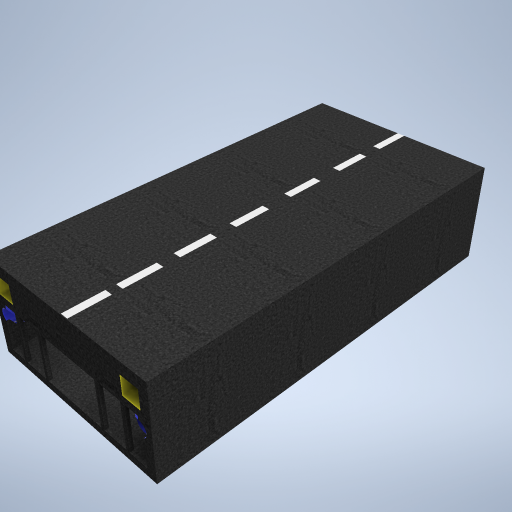
# Autodesk Inventor part: PLASTIC ROAD
Saved by Autodesk Inventor 2024 (Build 280153020, 153B)
## iProperties
Created: 2024-05-01
Part Number: PLASTIC ROAD
Material: Generic
Document SubType Name: Modeling
Designer: c7473124
Density: 1 g/cm^3
Appearance: Asphalt 2
Author: c7473124
Autodesk Inventor part; units mm, degrees
ref_plane "YZ Plane" through (0, 0, 0) normal (1, 0, 0) x (0, 1, 0)
ref_plane "XZ Plane" through (0, 0, 0) normal (0, 1, 0) x (-1, 0, 0)
ref_plane "XY Plane" through (0, 0, 0) normal (0, 0, 1) x (1, 0, 0)
sketch "Sketch1" plane through (0, 0, 0) normal (0, 0, 1) x (1, 0, 0)
  line L0 (0, 0) -> (1000, 0)
  line L1 (1000, 0) -> (1000, 500)
  line L2 (1000, 500) -> (0, 500)
  line L3 (0, 500) -> (0, 0)
  dimension "d0" = 1000
  dimension "d1" = 500
  constraints: 8 end point, 2 parallel, 1 horizontal, 1 perpendicular
  measures "d0" distance of L2.end L1.end
  measures "d1" distance of L1.end L0.end
extrude "Extrusion1" add sketch "Sketch1" along normal blind 2000
sketch "Sketch2" plane through (0, 0, 2000) normal (0, 0, 1) x (1, 0, 0)
  line L0 (947.5986, 433.5558) -> (847.5986, 433.5558)
  line L1 (847.5986, 433.5558) -> (847.5986, 333.5558)
  line L2 (847.5986, 333.5558) -> (947.5986, 333.5558)
  line L3 (947.5986, 333.5558) -> (947.5986, 433.5558)
  point P0 (0, 0)
  dimension "d4" = 100
  dimension "d5" = 100
  constraints: 8 end point, 2 parallel, 1 horizontal, 1 perpendicular
  measures "d4" distance of L2.end L1.end
  measures "d5" distance of L1.end L0.end
extrude "Extrusion2" cut sketch "Sketch2" against normal through all
sketch "Sketch3" plane through (0, 0, 2000) normal (0, 0, 1) x (1, 0, 0)
  line L0 (43.9995, 435.7022) -> (143.9995, 435.7022)
  line L1 (143.9995, 435.7022) -> (143.9995, 335.7022)
  line L2 (143.9995, 335.7022) -> (43.9995, 335.7022)
  line L3 (43.9995, 335.7022) -> (43.9995, 435.7022)
  point P0 (0, 0)
  dimension "d8" = 100
  dimension "d9" = 100
  constraints: 8 end point, 2 parallel, 1 horizontal, 1 perpendicular
  measures "d8" distance of L1.end L2.end
  measures "d9" distance of L0.end L1.end
extrude "Extrusion3" cut sketch "Sketch3" against normal through all
sketch "Sketch4" plane through (0, 0, 2000) normal (0, 0, 1) x (1, 0, 0)
  line L0 (50.4384, 294.0453) -> (949.7449, 294.0453)
  line L1 (949.7449, 294.0453) -> (949.7449, 42.9263)
  line L2 (949.7449, 42.9263) -> (50.4384, 42.9263)
  line L3 (50.4384, 42.9263) -> (50.4384, 294.0453)
  point P0 (0, 0)
  constraints: 8 end point, 2 parallel, 1 horizontal, 1 perpendicular
extrude "Extrusion4" cut sketch "Sketch4" against normal through all
sketch "Sketch5" plane through (50.4384, 42.9263, 2000) normal (1, 0, 0) x (0, 0, -1)
  line L0 (0, 251.119) -> (2000, 251.119) projected
  line L1 (2000, 251.119) -> (0, 251.119)
  line L2 (0, 251.119) -> (0, 171.119)
  line L3 (0, 171.119) -> (2000, 171.119)
  line L4 (2000, 171.119) -> (2000, 251.119)
  point P0 (2000, -42.9263)
  dimension "d14" = 2000
  dimension "d15" = 80
  constraints: 8 end point, 2 parallel, 1 horizontal, 1 perpendicular
  measures "d14" distance of L3.end L2.end
  measures "d15" distance of L2.end L1.end
extrude "Extrusion5" add sketch "Sketch5" along normal blind 70.5
sketch "Sketch6" plane through (0, 0, 2000) normal (0, 0, 1) x (1, 0, 0)
  line L0 (120.9384, 214.0453) -> (50.4384, 214.0453)
  line L1 (50.4384, 214.0453) -> (50.4384, 294.0453)
  line L2 (50.4384, 294.0453) -> (120.9384, 294.0453)
  line L3 (120.9384, 294.0453) -> (120.9384, 214.0453)
  point P0 (0, 0)
  constraints: 8 end point, 2 parallel, 1 horizontal, 1 perpendicular
extrude "Extrusion6" cut sketch "Sketch6" against normal through all
sketch "Sketch7" plane through (50.4384, 42.9263, 2000) normal (1, 0, 0) x (0, 0, -1)
  line L0 (0, 251.119) -> (2000, 251.119) projected
  line L1 (2000, 251.119) -> (0, 251.119)
  line L2 (0, 251.119) -> (0, 141.119)
  line L3 (0, 141.119) -> (2000, 141.119)
  line L4 (2000, 141.119) -> (2000, 251.119)
  point P0 (2000, -42.9263)
  dimension "d20" = 2000
  dimension "d21" = 110
  constraints: 8 end point, 2 parallel, 1 horizontal, 1 perpendicular
  measures "d20" distance of L3.end L2.end
  measures "d21" distance of L2.end L1.end
extrude "Extrusion7" add sketch "Sketch7" along normal blind 72
fillet "Fillet1" radius 50 3 edges at (122.4384, 239.0453, 2000) (86.4384, 184.0453, 2000) (122.4384, 184.0453, 1000)
sketch "Sketch8" plane through (0, 0, 2000) normal (0, 0, 1) x (1, 0, 0)
  line L0 (122.4384, 234.0453) -> (72.4384, 234.0453) projected
  circle A0 centre (72.4384, 234.0453) radius 40.25
  point P0 (0, 0)
  dimension "d25" = 80.5
  constraints: 1 centre point
  measures "d25" diameter of A0
extrude "Extrusion8" cut sketch "Sketch8" against normal through all
sketch "Sketch9" plane through (949.7449, 42.9263, 2000) normal (-1, 0, 0) x (0, 0, 1)
  line L0 (-50, 251.119) -> (-2000, 251.119) projected
  line L1 (-2000, 251.119) -> (0, 251.119)
  line L2 (0, 251.119) -> (0, 141.119)
  line L3 (0, 141.119) -> (-2000, 141.119)
  line L4 (-2000, 141.119) -> (-2000, 251.119)
  point P0 (-2000, -42.9263)
  dimension "d28" = 2000
  dimension "d29" = 110
  constraints: 8 end point, 2 parallel, 1 horizontal, 1 perpendicular
  measures "d28" distance of L2.end L3.end
  measures "d29" distance of L1.end L2.end
extrude "Extrusion9" add sketch "Sketch9" along normal blind 72
fillet "Fillet2" radius 50 3 edges at (877.7449, 239.0453, 2000) (913.7449, 184.0453, 2000) (877.7449, 184.0453, 1000)
sketch "Sketch10" plane through (0, 0, 2000) normal (0, 0, 1) x (1, 0, 0)
  line L0 (927.7449, 234.0453) -> (927.7449, 294.0453) projected
  circle A0 centre (927.7449, 234.0453) radius 41
  point P0 (0, 0)
  dimension "d33" = 82
  constraints: 1 centre point
  measures "d33" diameter of A0
extrude "Extrusion10" cut sketch "Sketch10" against normal through all
sketch "Sketch11" plane through (50.4384, 42.9263, 2000) normal (0, 1, 0) x (1, 0, 0)
  line L0 (93.5611, 0) -> (93.5611, 2000) projected
  line L1 (93.5611, 2000) -> (113.5611, 2000)
  line L2 (113.5611, 2000) -> (113.5611, 1980)
  line L3 (113.5611, 1980) -> (93.5611, 1980)
  line L4 (93.5611, 1980) -> (93.5611, 2000)
  point P0 (-50.4384, 2000)
  dimension "d36" = 20
  dimension "d37" = 20
  constraints: 8 end point, 2 parallel, 1 horizontal, 1 perpendicular
  measures "d36" distance of L2.end L3.end
  measures "d37" distance of L1.end L2.end
extrude "Extrusion11" add sketch "Sketch11" along normal through all
sketch "Sketch12" plane through (50.4384, 42.9263, 2000) normal (0, 1, 0) x (1, 0, 0)
  line L0 (797.1601, 0) -> (797.1601, 2000) projected
  line L1 (797.1601, 2000) -> (777.1601, 2000)
  line L2 (777.1601, 2000) -> (777.1601, 1980)
  line L3 (777.1601, 1980) -> (797.1601, 1980)
  line L4 (797.1601, 1980) -> (797.1601, 2000)
  point P0 (-50.4384, 2000)
  dimension "d40" = 20
  dimension "d41" = 20
  constraints: 8 end point, 2 parallel, 1 horizontal, 1 perpendicular
  measures "d40" distance of L3.end L2.end
  measures "d41" distance of L2.end L1.end
extrude "Extrusion12" add sketch "Sketch12" along normal through all
sketch "Sketch13" plane through (50.4384, 42.9263, 2000) normal (0, 1, 0) x (1, 0, 0)
  line L0 (777.1601, 2000) -> (113.5611, 2000) projected
  line L1 (258.2536, 2000) -> (278.2536, 2000)
  line L2 (278.2536, 2000) -> (278.2536, 1980)
  line L3 (278.2536, 1980) -> (258.2536, 1980)
  line L4 (258.2536, 1980) -> (258.2536, 2000)
  point P0 (-50.4384, 2000)
  dimension "d44" = 20
  dimension "d45" = 20
  constraints: 8 end point, 2 parallel, 1 horizontal, 1 perpendicular, 1 point on line
  measures "d44" distance of L2.end L3.end
  measures "d45" distance of L1.end L2.end
extrude "Extrusion13" add sketch "Sketch13" along normal through all
sketch "Sketch14" plane through (50.4384, 42.9263, 2000) normal (0, 1, 0) x (1, 0, 0)
  line L0 (278.2536, 2000) -> (777.1601, 2000) projected
  line L1 (651.9226, 2000) -> (631.9226, 2000)
  line L2 (631.9226, 2000) -> (631.9226, 1980)
  line L3 (631.9226, 1980) -> (651.9226, 1980)
  line L4 (651.9226, 1980) -> (651.9226, 2000)
  point P0 (-50.4384, 2000)
  dimension "d48" = 20
  dimension "d49" = 20
  constraints: 8 end point, 2 parallel, 1 horizontal, 1 perpendicular, 1 point on line
  measures "d48" distance of L3.end L2.end
  measures "d49" distance of L2.end L1.end
extrude "Extrusion14" add sketch "Sketch14" along normal through all
sketch "Sketch15" plane through (50.4384, 42.9263, 2000) normal (0, 1, 0) x (1, 0, 0)
  line L0 (93.5611, 0) -> (93.5611, 2000) projected
  line L1 (93.5611, 0) -> (113.5611, 0)
  line L2 (113.5611, 0) -> (113.5611, 20)
  line L3 (113.5611, 20) -> (93.5611, 20)
  line L4 (93.5611, 20) -> (93.5611, 0)
  point P0 (-50.4384, 2000)
  dimension "d52" = 20
  dimension "d53" = 20
  constraints: 8 end point, 2 parallel, 1 horizontal, 1 perpendicular
  measures "d52" distance of L3.end L2.end
  measures "d53" distance of L2.end L1.end
extrude "Extrusion15" add sketch "Sketch15" along normal through all
sketch "Sketch16" plane through (949.7449, 42.9263, 2000) normal (0, 1, 0) x (1, 0, 0)
  line L0 (-102.1463, 0) -> (-102.1463, 2000) projected
  line L1 (-102.1463, 0) -> (-122.1463, 0)
  line L2 (-122.1463, 0) -> (-122.1463, 20)
  line L3 (-122.1463, 20) -> (-102.1463, 20)
  line L4 (-102.1463, 20) -> (-102.1463, 0)
  point P0 (-949.7449, 2000)
  dimension "d56" = 20
  dimension "d57" = 20
  constraints: 8 end point, 2 parallel, 1 horizontal, 1 perpendicular
  measures "d56" distance of L2.end L3.end
  measures "d57" distance of L1.end L2.end
extrude "Extrusion16" add sketch "Sketch16" along normal through all
sketch "Sketch17" plane through (949.7449, 42.9263, 2000) normal (0, 1, 0) x (1, 0, 0)
  line L0 (-122.1463, 0) -> (-785.7454, 0) projected
  line L1 (-649.0702, 0) -> (-629.0702, 0)
  line L2 (-629.0702, 0) -> (-629.0702, 20)
  line L3 (-629.0702, 20) -> (-649.0702, 20)
  line L4 (-649.0702, 20) -> (-649.0702, 0)
  point P0 (-949.7449, 2000)
  dimension "d60" = 20
  dimension "d61" = 20
  constraints: 8 end point, 2 parallel, 1 horizontal, 1 perpendicular, 1 point on line
  measures "d60" distance of L3.end L2.end
  measures "d61" distance of L2.end L1.end
extrude "Extrusion17" add sketch "Sketch17" along normal through all
sketch "Sketch18" plane through (949.7449, 42.9263, 2000) normal (0, 1, 0) x (1, 0, 0)
  line L0 (-949.7449, 0) -> (50.2551, 0) projected
  line L1 (-254.9087, 0) -> (-274.9087, 0)
  line L2 (-274.9087, 0) -> (-274.9087, 20)
  line L3 (-274.9087, 20) -> (-254.9087, 20)
  line L4 (-254.9087, 20) -> (-254.9087, 0)
  point P0 (-949.7449, 2000)
  dimension "d64" = 20
  dimension "d65" = 20
  constraints: 8 end point, 2 parallel, 1 horizontal, 1 perpendicular, 1 point on line
  measures "d64" distance of L2.end L3.end
  measures "d65" distance of L1.end L2.end
extrude "Extrusion18" add sketch "Sketch18" along normal through all
sketch "Sketch19" plane through (949.7449, 42.9263, 2000) normal (0, 1, 0) x (1, 0, 0)
  line L0 (-529.2542, 439.7202) -> (-449.2542, 439.7202)
  line L1 (-449.2542, 439.7202) -> (-449.2542, 359.7202)
  line L2 (-449.2542, 359.7202) -> (-529.2542, 359.7202)
  line L3 (-529.2542, 359.7202) -> (-529.2542, 439.7202)
  point P0 (-949.7449, 2000)
  dimension "d68" = 80
  dimension "d69" = 80
  constraints: 8 end point, 2 parallel, 1 horizontal, 1 perpendicular
  measures "d68" distance of L1.end L2.end
  measures "d69" distance of L0.end L1.end
extrude "Extrusion19" add sketch "Sketch19" along normal through all
sketch "Sketch20" plane through (949.7449, 42.9263, 2000) normal (0, 1, 0) x (1, 0, 0)
  line L0 (-506.3949, 1061.6477) -> (-426.3949, 1061.6477)
  line L1 (-426.3949, 1061.6477) -> (-426.3949, 981.6477)
  line L2 (-426.3949, 981.6477) -> (-506.3949, 981.6477)
  line L3 (-506.3949, 981.6477) -> (-506.3949, 1061.6477)
  point P0 (-949.7449, 2000)
  dimension "d72" = 80
  dimension "d73" = 80
  constraints: 8 end point, 2 parallel, 1 horizontal, 1 perpendicular
  measures "d72" distance of L1.end L2.end
  measures "d73" distance of L0.end L1.end
extrude "Extrusion20" add sketch "Sketch20" along normal through all
sketch "Sketch21" plane through (949.7449, 42.9263, 2000) normal (0, 1, 0) x (1, 0, 0)
  line L0 (-420.7918, 1427.5421) -> (-500.7918, 1427.5421)
  line L1 (-500.7918, 1427.5421) -> (-500.7918, 1507.5421)
  line L2 (-500.7918, 1507.5421) -> (-420.7918, 1507.5421)
  line L3 (-420.7918, 1507.5421) -> (-420.7918, 1427.5421)
  point P0 (-949.7449, 2000)
  dimension "d76" = 80
  dimension "d77" = 80
  constraints: 8 end point, 2 parallel, 1 horizontal, 1 perpendicular
  measures "d76" distance of L1.end L2.end
  measures "d77" distance of L0.end L1.end
extrude "Extrusion21" add sketch "Sketch21" along normal through all
sketch "Sketch22" plane through (949.7449, 42.9263, 2000) normal (0, 1, 0) x (1, 0, 0)
  circle A0 centre (-203.7916, 715.5889) radius 25
  point P0 (-949.7449, 2000)
  dimension "d80" = 50
  constraints: 1 centre point
  measures "d80" diameter of A0
extrude "Extrusion22" add sketch "Sketch22" along normal blind 20
sketch "Sketch23" plane through (949.7449, 42.9263, 2000) normal (0, 1, 0) x (1, 0, 0)
  circle A0 centre (-699.6316, 699.2521) radius 25
  point P0 (-949.7449, 2000)
  dimension "d83" = 50
  constraints: 1 centre point
  measures "d83" diameter of A0
extrude "Extrusion23" add sketch "Sketch23" along normal blind 20
sketch "Sketch24" plane through (949.7449, 42.9263, 2000) normal (0, 1, 0) x (1, 0, 0)
  circle A0 centre (-711.9582, 1376.1969) radius 25
  point P0 (-949.7449, 2000)
  dimension "d86" = 50
  constraints: 1 centre point
  measures "d86" diameter of A0
extrude "Extrusion24" add sketch "Sketch24" along normal blind 20
sketch "Sketch25" plane through (949.7449, 42.9263, 2000) normal (0, 1, 0) x (1, 0, 0)
  circle A0 centre (-187.3173, 1236.8057) radius 25
  point P0 (-949.7449, 2000)
  dimension "d89" = 50
  constraints: 1 centre point
  measures "d89" diameter of A0
extrude "Extrusion25" add sketch "Sketch25" along normal blind 20
sketch "Sketch26" plane through (0, 500, 0) normal (0, 1, 0) x (1, 0, 0)
  line L0 (0, 0) -> (1000, 0) projected
  line L1 (500, 0) -> (540, 0)
  line L2 (540, 0) -> (540, -196)
  line L3 (540, -196) -> (500, -196)
  line L4 (500, -196) -> (500, 0)
  dimension "d92" = 40
  dimension "d93" = 196
  constraints: 8 end point, 2 parallel, 1 horizontal, 1 midpoint, 1 perpendicular
  measures "d92" distance of L2.end L3.end
  measures "d93" distance of L1.end L2.end
extrude "Extrusion26" add sketch "Sketch26" along normal blind 0.001
sketch "Sketch27" plane through (2.2498, 500, 301.4963) normal (0, 1, 0) x (1, 0, 0)
  line L0 (0, 0) -> (1000, 0)
  line L1 (500, 0) -> (540, 0)
  line L2 (540, 0) -> (540, -196)
  line L3 (540, -196) -> (500, -196)
  line L4 (500, -196) -> (500, 0)
  dimension "d96" = 40
  dimension "d97" = 196
  constraints: 10 end point, 2 parallel, 1 horizontal, 1 midpoint, 1 perpendicular
  measures "d96" distance of L2.end L3.end
  measures "d97" distance of L1.end L2.end
extrude "Extrusion27" add sketch "Sketch27" along normal blind 0.001
sketch "Sketch28" plane through (1.351, 500, 629.1001) normal (0, 1, 0) x (1, 0, 0)
  line L0 (0, 0) -> (1000, 0)
  line L1 (500, 0) -> (540, 0)
  line L2 (540, 0) -> (540, -196)
  line L3 (540, -196) -> (500, -196)
  line L4 (500, -196) -> (500, 0)
  dimension "d101" = 40
  dimension "d102" = 196
  constraints: 10 end point, 2 parallel, 1 horizontal, 1 midpoint, 1 perpendicular
  measures "d101" distance of L2.end L3.end
  measures "d102" distance of L1.end L2.end
extrude "Extrusion28" add sketch "Sketch28" along normal blind 0.001
sketch "Sketch29" plane through (5.006, 500, 965.1502) normal (0, 1, 0) x (1, 0, 0)
  line L0 (0, 0) -> (1000, 0)
  line L1 (500, 0) -> (540, 0)
  line L2 (540, 0) -> (540, -196)
  line L3 (540, -196) -> (500, -196)
  line L4 (500, -196) -> (500, 0)
  dimension "d106" = 40
  dimension "d107" = 196
  constraints: 10 end point, 2 parallel, 1 horizontal, 1 midpoint, 1 perpendicular
  measures "d106" distance of L2.end L3.end
  measures "d107" distance of L1.end L2.end
extrude "Extrusion29" add sketch "Sketch29" along normal blind 0.001
sketch "Sketch30" plane through (6.1364, 500, 1270.3317) normal (0, 1, 0) x (1, 0, 0)
  line L0 (0, 0) -> (1000, 0)
  line L1 (500, 0) -> (540, 0)
  line L2 (540, 0) -> (540, -196)
  line L3 (540, -196) -> (500, -196)
  line L4 (500, -196) -> (500, 0)
  dimension "d111" = 40
  dimension "d112" = 196
  constraints: 10 end point, 2 parallel, 1 horizontal, 1 midpoint, 1 perpendicular
  measures "d111" distance of L2.end L3.end
  measures "d112" distance of L1.end L2.end
extrude "Extrusion30" add sketch "Sketch30" along normal blind 0.001
sketch "Sketch31" plane through (8.9477, 500, 1554.2732) normal (0, 1, 0) x (1, 0, 0)
  line L0 (0, 0) -> (1000, 0)
  line L1 (500, 0) -> (540, 0)
  line L2 (540, 0) -> (540, -196)
  line L3 (540, -196) -> (500, -196)
  line L4 (500, -196) -> (500, 0)
  dimension "d116" = 40
  dimension "d117" = 196
  constraints: 10 end point, 2 parallel, 1 horizontal, 1 midpoint, 1 perpendicular
  measures "d116" distance of L2.end L3.end
  measures "d117" distance of L1.end L2.end
extrude "Extrusion31" add sketch "Sketch31" along normal blind 0.001
sketch "Sketch32" plane through (8.7391, 500, 1799.6878) normal (0, 1, 0) x (1, 0, 0)
  line L0 (0, 0) -> (1000, 0)
  line L1 (500, 0) -> (540, 0)
  line L2 (540, 0) -> (540, -196)
  line L3 (540, -196) -> (500, -196)
  line L4 (500, -196) -> (500, 0)
  dimension "d121" = 40
  dimension "d122" = 196
  constraints: 10 end point, 2 parallel, 1 horizontal, 1 midpoint, 1 perpendicular
  measures "d121" distance of L2.end L3.end
  measures "d122" distance of L1.end L2.end
extrude "Extrusion32" add sketch "Sketch32" along normal blind 0.001
body "Solid1"
